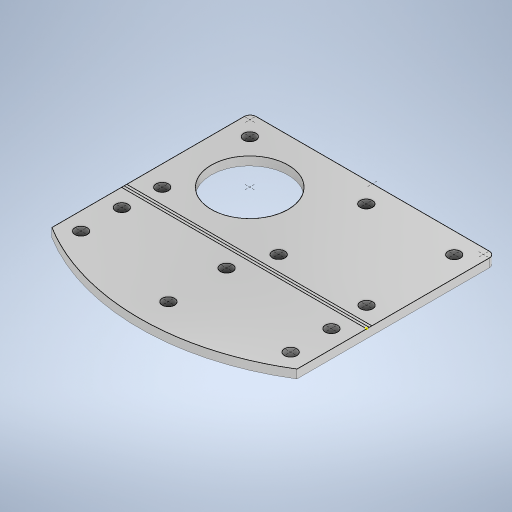
# Autodesk Inventor part: axis_2_bottom_L_frame(bottom)
Saved by Autodesk Inventor 2024.2 (Build 282272000, 272)
## iProperties
Created: 2023-12-25
Part Number: axis_2_bottom_L_frame(bottom)
Material: Aluminum 6061-AHC
Document SubType Name: Modeling
Designer: chanh
Density: 2.7 g/cm^3
Appearance: Aluminum - Dark
Author: chanh
Autodesk Inventor part; units mm, degrees
ref_plane "YZ Plane" through (0, 0, 0) normal (1, 0, 0) x (0, 1, 0)
ref_plane "XZ Plane" through (0, 0, 0) normal (0, 1, 0) x (-1, 0, 0)
ref_plane "XY Plane" through (0, 0, 0) normal (0, 0, 1) x (1, 0, 0)
sketch "Sketch1" plane through (0, 0, 0) normal (0, 1, 0) x (-1, 0, 0)
  line L0 (42.1, -0.4496) -> (0, -0.4496)
  circle A0 centre (3.05, 10) radius 1.05
  circle A1 centre (3.05, 3) radius 1.05
  circle A2 centre (21.05, 3) radius 1.05
  circle A3 centre (21.05, 13) radius 1.05
  circle A4 centre (39.05, 10) radius 1.05
  circle A5 centre (39.05, 3) radius 1.05
  circle A6 centre (3.5, -18.5443) radius 1.05
  circle A7 centre (18.6, -18.5443) radius 1.05
  circle A8 centre (38.6, -18.5443) radius 1.05
  circle A9 centre (38.6, -3.4943) radius 1.05
  circle A10 centre (18.6, -3.4943) radius 1.05
  circle A11 centre (3.5, -3.4943) radius 1.05
  circle A12 centre (31.1, -11.0193) radius 6.6
  arc A13 (41.1, -22.0893) -> (42.1, -21.0893) centre (41.1, -21.0893) ccw
  line L1 (41.1, -22.0893) -> (1, -22.0893)
  arc A14 (0, -21.0893) -> (1, -22.0893) centre (1, -21.0893) ccw
  arc A15 (42.1, 11.9532) -> (0, 11.9532) centre (21.05, -22.06) ccw
  line L2 (0, -21.0893) -> (0, 11.9532)
  line L3 (42.1, 11.9532) -> (42.1, -21.0893)
  line L4 (42.1, -0.8993) -> (0, -0.8993)
  line L5 (0, 0) -> (42.1, 0)
  constraints: 16 centre point, 12 end point, 6 point on circle, 6 point on line, 4 horizontal, 2 vertical, 45 other
extrude "Extrusion1" add sketch "Sketch1" against normal blind 1.5
body "Solid1"
